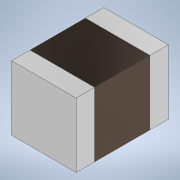
# Autodesk Inventor part: Part3
Saved by Autodesk Inventor 2021 (Build 250183000, 183)
## iProperties
Created: 2023-04-01
Part Number: Part3
Material: Generic
Document SubType Name: Modeling
Designer: stepa
Density: 1 g/cm^3
Appearance: Default
Author: stepa
Autodesk Inventor part; units mm, degrees
ref_plane "YZ Plane" through (0, 0, 0) normal (1, 0, 0) x (0, 1, 0)
ref_plane "XZ Plane" through (0, 0, 0) normal (0, 1, 0) x (-1, 0, 0)
ref_plane "XY Plane" through (0, 0, 0) normal (0, 0, 1) x (1, 0, 0)
sketch "Sketch1" plane through (0, 0, 0) normal (0, 0, 1) x (1, 0, 0)
  line L0 (-0.7, 0.7) -> (0.7, 0.7)
  line L1 (0.7, 0.7) -> (0.7, -0.7)
  line L2 (0.7, -0.7) -> (-0.7, -0.7)
  line L3 (-0.7, -0.7) -> (-0.7, 0.7)
  line L4 (-0.7, 0.7) -> (0.7, -0.7) construction
  line L5 (0.7, 0.7) -> (-0.7, -0.7) construction
  point P0 (0, 0)
  dimension "d0" = 1.4
  dimension "d1" = 1.4
  constraints: 12 end point, 2 midpoint, 2 parallel, 1 horizontal, 1 perpendicular
  measures "d0" distance of L0.end L1.end
  measures "d1" distance between parallel lines of L1 L3
extrude "Extrusion1" add sketch "Sketch1" along normal mid plane 1.2
sketch "Sketch2" plane through (0, 0, 0.6) normal (0, 0, 1) x (1, 0, 0)
  line L0 (-0.7, -0.7) -> (0.7, -0.7) projected
  line L1 (0.7, -0.7) -> (0.7, 0.7) projected
  line L2 (0.7, 0.7) -> (-0.7, 0.7) projected
  line L3 (-0.7, 0.7) -> (-0.7, -0.7) projected
  point P0 (0, 0)
extrude "Extrusion2" add sketch "Sketch2" along normal blind 0.4 separate body
mirror "Mirror1" about plane through (0, 0, 0) normal (0, 0, 1) of "Extrusion2" bodies 2
body "Solid1"
body "Solid2"
